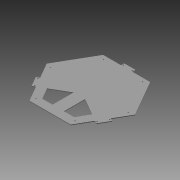
# Autodesk Inventor part: base_constr
Saved by Autodesk Inventor 2015 (Build 190159000, 159)
## iProperties
Created: 2015-04-17
Part Number: base_constr
Material: Ogólny
Document SubType Name: Modeling
Designer: Marcin
Density: 1 g/cm^3
Appearance: Domyślna
Author: Marcin
Autodesk Inventor part; units mm, degrees
ref_plane "YZ Plane" through (0, 0, 0) normal (1, 0, 0) x (0, 1, 0)
ref_plane "XZ Plane" through (0, 0, 0) normal (0, 1, 0) x (-1, 0, 0)
ref_plane "XY Plane" through (0, 0, 0) normal (0, 0, 1) x (1, 0, 0)
sketch "Szkic1" plane through (0, 0, 0) normal (0, 0, 1) x (1, 0, 0)
  line L0 (17.5, 0) -> (-17.5, 0)
  line L1 (-17.5, 0) -> (-17.5, 125)
  line L2 (-17.5, 125) -> (17.5, 125)
  line L3 (17.5, 125) -> (17.5, 0)
  line L4 (0, 0) -> (0, 163.4249) construction
  line L5 (-8.75, 15.1554) -> (8.75, -15.1554)
  line L6 (8.75, -15.1554) -> (-99.5032, -77.6554)
  line L7 (-99.5032, -77.6554) -> (-117.0032, -47.3446)
  line L8 (-117.0032, -47.3446) -> (-8.75, 15.1554)
  line L9 (0, 0) -> (-141.5301, -81.7124) construction
  line L10 (-8.75, -15.1554) -> (8.75, 15.1554)
  line L11 (8.75, 15.1554) -> (117.0032, -47.3446)
  line L12 (117.0032, -47.3446) -> (99.5032, -77.6554)
  line L13 (99.5032, -77.6554) -> (-8.75, -15.1554)
  line L14 (0, 0) -> (141.5301, -81.7124) construction
  dimension "d0" = 125
  dimension "d1" = 35
  dimension "d4" = 360
  constraints: 30 end point, 3 midpoint, 2 coincident, 2 parallel, 1 horizontal, 1 perpendicular, 1 vertical, 33 other
  measures "d0" distance of L2.end L0.start
  measures "d1" distance of L1.end L2.end
extrude "Wyciągnięcie proste1" add sketch "Szkic1" along normal blind 2
sketch "Szkic3" plane through (0, 0, 0) normal (0, 0, -1) x (-1, 0, 0)
  line L0 (-99.5032, -77.6554) -> (0, -20.2073) projected
  line L1 (0, -20.2073) -> (99.5032, -77.6554) projected
  line L2 (0, -20.2073) -> (0, -155.6549) construction
  line L3 (-90.9327, -72.7073) -> (-63.5085, -120.2073)
  line L4 (-63.5085, -120.2073) -> (0, -120.2073)
  line L5 (-49.0748, -95.2073) -> (0, -95.2073)
  line L6 (-49.0748, -95.2073) -> (-69.282, -60.2073)
  line L7 (90.9327, -72.7073) -> (63.5085, -120.2073)
  line L8 (63.5085, -120.2073) -> (0, -120.2073)
  line L9 (49.0748, -95.2073) -> (0, -95.2073)
  line L10 (49.0748, -95.2073) -> (69.282, -60.2073)
  line L11 (90.9327, -72.7073) -> (69.282, -60.2073)
  line L12 (-90.9327, -72.7073) -> (-69.282, -60.2073)
  point P0 (0, 0)
  dimension "d12" = 25
  dimension "d15" = 25
  dimension "d16" = 80
  dimension "d17" = 75
  constraints: 22 end point, 4 point on line, 4 symmetric about line, 2 perpendicular, 1 collinear, 1 horizontal, 1 parallel
  measures "d12" distance between parallel lines of L5 L4
  measures "d15" distance between parallel lines of L6 L3
  measures "d16" distance of L0.end L6.end
  measures "d17" distance of L0.end L5.end
extrude "Wyciągnięcie proste3" add sketch "Szkic3" against normal blind 2 contours L0 L6 L5 L9 L10 L1 L7 L8 L4 L3
sketch "Szkic5" plane through (0, 0, 2) normal (0, 0, 1) x (1, 0, 0)
  line L0 (-49.0748, -95.2073) -> (-69.282, -60.2073) projected
  line L1 (69.282, -60.2073) -> (49.0748, -95.2073) projected
  line L2 (-69.282, -60.2073) -> (0, -20.2073)
  line L3 (0, -20.2073) -> (69.282, -60.2073)
  line L4 (69.282, -60.2073) -> (49.0748, -95.2073)
  line L5 (-49.0748, -95.2073) -> (-69.282, -60.2073)
  line L6 (-90.9327, -72.7073) -> (-63.5085, -120.2073) projected
  line L7 (-63.5085, -120.2073) -> (63.5085, -120.2073) projected
  line L8 (63.5085, -120.2073) -> (90.9327, -72.7073) projected
  line L9 (-90.9327, -72.7073) -> (-63.5085, -120.2073)
  line L10 (63.5085, -120.2073) -> (-63.5085, -120.2073)
  line L11 (90.9327, -72.7073) -> (63.5085, -120.2073)
  line L12 (90.9327, -72.7073) -> (99.5032, -77.6554) projected
  line L13 (86.782, -29.8964) -> (17.5, 10.1036)
  line L14 (17.5, 10.1036) -> (17.5, 90.1036)
  line L15 (17.5, 90.1036) -> (57.9145, 90.1036)
  line L16 (106.9893, 5.1036) -> (86.782, -29.8964)
  line L17 (108.4327, -42.3964) -> (135.8568, 5.1036)
  line L18 (72.3483, 115.1036) -> (135.8568, 5.1036)
  line L19 (17.5, 115.1036) -> (72.3483, 115.1036)
  line L20 (-17.5, 90.1036) -> (-17.5, 10.1036)
  line L21 (-17.5, 10.1036) -> (-86.782, -29.8964)
  line L22 (-86.782, -29.8964) -> (-106.9893, 5.1036)
  line L23 (-57.9145, 90.1036) -> (-17.5, 90.1036)
  line L24 (-17.5, 115.1036) -> (-72.3483, 115.1036)
  line L25 (-135.8568, 5.1036) -> (-72.3483, 115.1036)
  line L26 (-108.4327, -42.3964) -> (-135.8568, 5.1036)
  line L27 (-106.9893, 5.1036) -> (-57.9145, 90.1036)
  line L28 (106.9893, 5.1036) -> (57.9145, 90.1036)
  line L29 (-108.4327, -42.3964) -> (-86.782, -29.8964)
  line L30 (-117.0032, -47.3446) -> (-17.5, 10.1036) projected
  line L31 (108.4327, -42.3964) -> (86.782, -29.8964)
  line L32 (17.5, 10.1036) -> (117.0032, -47.3446) projected
  line L33 (17.5, 90.1036) -> (17.5, 115.1036)
  line L34 (17.5, 125) -> (17.5, 10.1036) projected
  line L35 (-17.5, 90.1036) -> (-17.5, 115.1036)
  line L36 (-17.5, 10.1036) -> (-17.5, 125) projected
  point P0 (0, 0)
  dimension "d24" = 360
  constraints: 54 end point, 6 collinear, 1 horizontal, 1 perpendicular, 49 other
extrude "Wyciągnięcie proste5" add sketch "Szkic5" against normal blind 2 contours L16 L28 L15 L33 L19 L18 L17 L31 | L23 L27 L22 L29 L26 L25 L24 L35
sketch "Szkic6" plane through (0, 0, 2) normal (0, 0, 1) x (1, 0, 0)
  line L0 (-63.5085, -120.2073) -> (63.5085, -120.2073) projected
  line L1 (17.5, 10.1036) -> (17.5, 90.1036) projected
  line L2 (-17.5, 90.1036) -> (-17.5, 10.1036) projected
  line L3 (17.5, 10.1036) -> (-17.5, 10.1036)
  line L4 (-17.5, 10.1036) -> (-17.5, -120.2073)
  line L5 (-17.5, -120.2073) -> (17.5, -120.2073)
  line L6 (17.5, -120.2073) -> (17.5, 10.1036)
  point P0 (0, 0)
  constraints: 8 end point, 2 parallel, 1 collinear, 1 horizontal, 1 perpendicular, 1 point on line
extrude "Wyciągnięcie proste6" add sketch "Szkic6" against normal blind 2
sketch "Szkic7" plane through (0, 0, 0) normal (0, 0, -1) x (-1, 0, 0)
  line L0 (0, 0) -> (60, 103.923) construction
  line L1 (0, 0) -> (0, 71.3252)
  point P0 (-60, 103.923)
  point P1 (-120, 0)
  point P2 (-60, -103.923)
  point P3 (60, -103.923)
  point P4 (120, 0)
  dimension "d30" = 120
  dimension "d33" = 360
  dimension "d42" = 30
  constraints: 4 end point, 1 coincident, 1 vertical, 7 other
  measures "d30" distance of L0.start L0.end
  measures "d42" angle of L0 L1
hole "Otwór1" at (-60, 103.923, 0) at (60, 103.923, 0) at (120, 0, 0) at (60, -103.923, 0) at (-60, -103.923, 0) at (-120, 0, 0) direction (0, 0, 1) diameter 3 depth 8 tip angle 118
sketch "Szkic8" plane through (0, 0, 0) normal (0, 0, -1) x (-1, 0, 0)
  point P0 (-96.057, -71.6244)
  point P1 (-110.057, -47.3756)
  point P2 (-14, 119)
  point P3 (14, 119)
  point P4 (110.057, -47.3756)
  point P5 (96.057, -71.6244)
hole "Otwór2" at (96.057, -71.6244, 0) at (110.057, -47.3756, 0) at (14, 119, 0) at (-14, 119, 0) at (-110.057, -47.3756, 0) at (-96.057, -71.6244, 0) direction (0, 0, 1) diameter 3.4 depth 2
sketch "Szkic9" plane through (0, 0, 0) normal (0, 0, -1) x (-1, 0, 0)
  circle A0 centre (110.057, -47.3756) radius 1.7 projected
  circle A1 centre (-14, 119) radius 1.7 projected
  circle A2 centre (-96.057, -71.6244) radius 1.7 projected
  circle A3 centre (-110.057, -47.3756) radius 1.7 projected
  circle A4 centre (14, 119) radius 1.7 projected
  circle A5 centre (96.057, -71.6244) radius 1.7 projected
  circle A6 centre (60, -103.923) radius 1.5 projected
  circle A7 centre (-120, 0) radius 1.5 projected
  circle A8 centre (60, 103.923) radius 1.5 projected
  circle A9 centre (-60, 103.923) radius 1.5 projected
  circle A10 centre (-60, -103.923) radius 1.5 projected
  circle A11 centre (120, 0) radius 1.5 projected
  line L0 (-17.5, -95.2073) -> (-49.0748, -95.2073) projected
  line L1 (-49.0748, -95.2073) -> (-69.282, -60.2073) projected
  line L2 (-69.282, -60.2073) -> (-17.5, -30.3109) projected
  line L3 (-17.5, -30.3109) -> (-17.5, -95.2073) projected
  line L4 (-63.5085, -120.2073) -> (63.5085, -120.2073) projected
  line L5 (63.5085, -120.2073) -> (90.9327, -72.7073) projected
  line L6 (90.9327, -72.7073) -> (99.5032, -77.6554) projected
  line L7 (99.5032, -77.6554) -> (117.0032, -47.3446) projected
  line L8 (117.0032, -47.3446) -> (108.4327, -42.3964) projected
  line L9 (108.4327, -42.3964) -> (135.8568, 5.1036) projected
  line L10 (135.8568, 5.1036) -> (72.3483, 115.1036) projected
  line L11 (72.3483, 115.1036) -> (17.5, 115.1036) projected
  line L12 (17.5, 115.1036) -> (17.5, 125) projected
  line L13 (17.5, 125) -> (-17.5, 125) projected
  line L14 (-17.5, 125) -> (-17.5, 115.1036) projected
  line L15 (-17.5, 115.1036) -> (-72.3483, 115.1036) projected
  line L16 (-72.3483, 115.1036) -> (-135.8568, 5.1036) projected
  line L17 (-135.8568, 5.1036) -> (-108.4327, -42.3964) projected
  line L18 (-108.4327, -42.3964) -> (-117.0032, -47.3446) projected
  line L19 (-117.0032, -47.3446) -> (-99.5032, -77.6554) projected
  line L20 (-99.5032, -77.6554) -> (-90.9327, -72.7073) projected
  line L21 (-90.9327, -72.7073) -> (-63.5085, -120.2073) projected
  line L22 (17.5, -95.2073) -> (17.5, -30.3109) projected
  line L23 (17.5, -30.3109) -> (69.282, -60.2073) projected
  line L24 (69.282, -60.2073) -> (49.0748, -95.2073) projected
  line L25 (49.0748, -95.2073) -> (17.5, -95.2073) projected
  line L26 (17.5, 10.1036) -> (17.5, 90.1036) projected
  line L27 (17.5, 90.1036) -> (57.9145, 90.1036) projected
  line L28 (57.9145, 90.1036) -> (106.9893, 5.1036) projected
  line L29 (106.9893, 5.1036) -> (86.782, -29.8964) projected
  line L30 (86.782, -29.8964) -> (17.5, 10.1036) projected
  line L31 (-17.5, 10.1036) -> (-86.782, -29.8964) projected
  line L32 (-86.782, -29.8964) -> (-106.9893, 5.1036) projected
  line L33 (-106.9893, 5.1036) -> (-57.9145, 90.1036) projected
  line L34 (-57.9145, 90.1036) -> (-17.5, 90.1036) projected
  line L35 (-17.5, 90.1036) -> (-17.5, 10.1036) projected
  line L36 (-106.9893, 5.1036) -> (-57.9145, 90.1036) projected
  point P0 (0, 0)
extrude "Wyciągnięcie proste7" add sketch "Szkic9" against normal blind 2 contours L26 L27 L28 L29 L30 | L31 L32 L33 L34 L35
